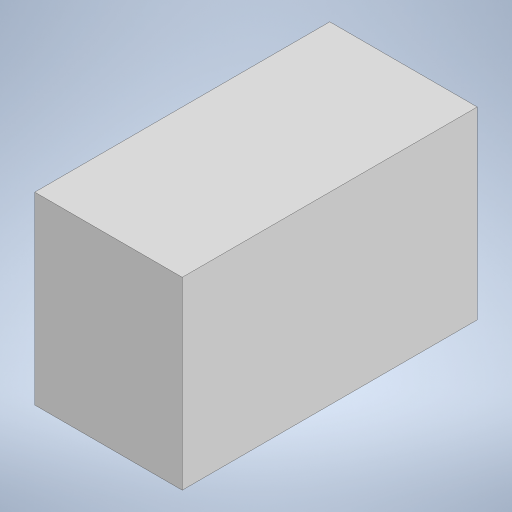
# Autodesk Inventor part: endcap_4mm_2ea_typeB_ver2_onyx
Saved by Autodesk Inventor 2024 (Build 280153000, 153)
## iProperties
Created: 2023-11-06
Part Number: endcap_4mm_2ea_typeB_ver2_onyx
Material: 일반
Document SubType Name: Modeling
Designer: Gihyeok Na
Density: 1 g/cm^3
Appearance: 기본값
Author: Gihyeok Na
Autodesk Inventor part; units mm, degrees
ref_plane "YZ Plane" through (0, 0, 0) normal (1, 0, 0) x (0, 1, 0)
ref_plane "XZ Plane" through (0, 0, 0) normal (0, 1, 0) x (-1, 0, 0)
ref_plane "XY Plane" through (0, 0, 0) normal (0, 0, 1) x (1, 0, 0)
sketch "스케치1" plane through (0, 0, 0) normal (0, 1, 0) x (-1, 0, 0)
  circle A0 centre (0, 0) radius 1.6
  circle A1 centre (0, 0) radius 2.4
  circle A2 centre (0, -4.8) radius 2.4
  circle A3 centre (0, -4.8) radius 1.6
  line L0 (1.6, 0) -> (1.6, -4.8)
  line L1 (-1.6, 0) -> (-1.6, -4.8)
  line L2 (-2.4, 2.4) -> (2.4, 2.4)
  line L3 (2.4, 2.4) -> (2.4, -7.2)
  line L4 (2.4, -7.2) -> (-2.4, -7.2)
  line L5 (-2.4, -7.2) -> (-2.4, 2.4)
  point P0 (0, -2.4)
  dimension "d1" = 4.8
  dimension "d2" = 4.8
  dimension "d0" = 3.2
  dimension "d3" = 3.2
  constraints: 12 end point, 4 point on circle, 3 coincident, 3 horizontal, 2 centre point, 2 parallel, 2 tangent, 2 vertical, 2 vertical alignment, 1 perpendicular, 4 other
  measures "d0" diameter of A0
  measures "d3" diameter of A3
extrude "돌출3" add sketch "스케치1" against normal blind 2 contours L0 A1 L1 A0 | A0 L1 A1 L0 | L0 A2 A1 | A1 L3 A2 L0 | L1 A2 L5 A1 | A1 A2 L1 | A2 L0 A3 L1 | A1 L2 L3 | A2 L1 A3 L0 | L5 L2 A1 | L3 L4 A2 | A2 L4 L5
extrude "돌출4" add sketch "스케치1" along normal blind 4 contours A0 L1 A1 L0 | A1 L3 A2 L0 | L1 A2 L5 A1 | A1 L2 L3 | A2 L1 A3 L0 | L5 L2 A1 | L3 L4 A2 | A2 L4 L5 picked at (-1.7127, -1.0681) picked at (-1.7127, -3.7319)
sketch "스케치2" plane through (0, 4, 0) normal (0, 1, 0) x (1, 0, 0)
  line L0 (-2.4, -2.4) -> (2.4, -2.4) projected
  line L1 (2.4, -2.4) -> (2.4, 7.2) projected
  line L2 (2.4, 7.2) -> (-2.4, 7.2) projected
  line L3 (-2.4, 7.2) -> (-2.4, -2.4) projected
  line L4 (-1.6, 0) -> (-1.6, 4.8) projected
  arc A0 (1.6, 4.8) -> (-1.6, 4.8) centre (0, 4.8) ccw projected
  line L5 (1.6, 4.8) -> (1.6, 0) projected
  arc A1 (-1.6, 0) -> (1.6, 0) centre (0, 0) ccw projected
extrude "돌출5" add sketch "스케치2" against normal blind 0.8 contours L3 L2 L1 L0 | L4 A0 L5 A1
sketch "스케치3" plane through (2.4, -2, -7.2) normal (0, 0, -1) x (-1, 0, 0)
  circle A0 centre (2.4, 3.6) radius 1.6
  line L0 (0, 6) -> (4.8, 6) projected
  circle A1 centre (2.4, 3.6) radius 2.4
  line L1 (4.8, 0) -> (4.8, 6) projected
  point P0 (2.4, 2)
  dimension "d14" = 3.2
  dimension "d15" = 2.4
  dimension "d16" = 4.8
  constraints: 2 centre point, 1 coincident, 1 tangent
  measures "d14" diameter of A0
  measures "d15" distance from line of L0 A0.centre
  measures "d16" diameter of A1
extrude "돌출6" cut sketch "스케치3" against normal blind 3.3 contours A0
